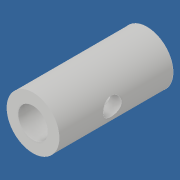
# Autodesk Inventor part: unThread insert
Saved by Autodesk Inventor 2018 (Build 220112000, 112)
## iProperties
Created: 2018-04-26
Part Number: unThread insert
Material: Generic
Document SubType Name: Modeling
Designer: 232963
Density: 1 g/cm^3
Appearance: Default
Author: 232963
Autodesk Inventor part; units mm, degrees
ref_plane "YZ Plane" through (0, 0, 0) normal (1, 0, 0) x (0, 1, 0)
ref_plane "XZ Plane" through (0, 0, 0) normal (0, 1, 0) x (-1, 0, 0)
ref_plane "XY Plane" through (0, 0, 0) normal (0, 0, 1) x (1, 0, 0)
sketch "Sketch1" plane through (0, 0, 0) normal (0, 0, 1) x (1, 0, 0)
  circle A0 centre (0, 0) radius 8.763
  circle A1 centre (0, 0) radius 5
  dimension "d0" = 17.526
  dimension "d1" = 10
  constraints: 2 centre point, 2 coincident
  measures "d0" diameter of A0
  measures "d1" diameter of A1
extrude "Extrusion1" add sketch "Sketch1" along normal blind 38.1
sketch "Sketch2" plane through (0, 0, 0) normal (1, 0, 0) x (0, 1, 0)
  line L0 (8.763, 38.1) -> (-8.763, 38.1) projected
  line L1 (-8.763, 0) -> (8.763, 0) projected
  line L2 (-5, 0) -> (-5, 38.1) projected
  line L3 (-8.763, 0) -> (-8.763, 38.1) projected
  line L4 (8.763, 0) -> (8.763, 38.1) projected
  circle A0 centre (0, 20.32) radius 3.0607
  point P0 (0, 0)
  dimension "d4" = 17.526
  dimension "d5" = 8.763
  dimension "d6" = 6.1214
  dimension "d7" = 20.32
  constraints: 1 centre point
  measures "d4" distance between parallel lines of L4 L3
  measures "d5" distance from line of L4 A0.centre
  measures "d6" diameter of A0
  measures "d7" distance from line of L1 A0.centre
extrude "Extrusion2" cut sketch "Sketch2" along normal mid plane 25.4 contours A0
body "Solid1"
